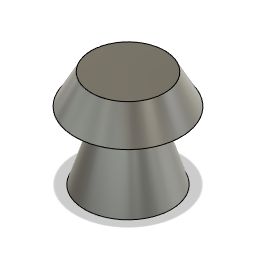
forme1 protopapier v1 (Autodesk Fusion 360 design; units mm, degrees)
Autodesk Fusion 360 part; units mm, degrees
sketch "Esquisse1" plane through (0, 0, 0) normal (0, 0, 1) x (1, 0, 0)
  line L0 (0, 0) -> (-65, 0)
  line L1 (-65, 0) -> (-40, 80)
  line L2 (-40, 80) -> (-79.5161, 101.5285)
  line L3 (-79.5161, 101.5285) -> (-55, 146.5285)
  line L4 (-55, 146.5285) -> (0, 146.8871)
  line L5 (0, 146.8871) -> (0, 0)
  dimension "d1" = 65
  dimension "d2" = 45
  dimension "d3" = 45
  dimension "d4" = 40
  dimension "d5" = 80
  dimension "d6" = 55
  constraint coincident L0.start L5.end
  constraint horizontal L0
  constraint perpendicular L2 L3
  constraint perpendicular L0 L5
  measures "d1" distance of L0.start L0.end
  measures "d2" distance of L1.end L2.end
  measures "d3" vertical distance of L2.end L3.end
  measures "d4" distance of L1.end L5
  measures "d5" vertical distance of L0.end L1.end
  measures "d6" horizontal distance of L3.end L4.end
revolve "Révolution1" add sketch "Esquisse1" angle 360 about axis through (0, 146.8871, 0) along (0, -1, 0)
shell "Coque1" thickness 2 removed faces 1 at (20.2416, 0, -0.2148)
